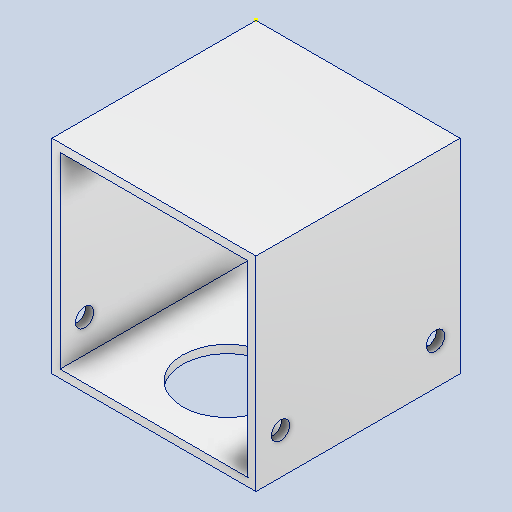
# Autodesk Inventor part: ankle
Saved by Autodesk Inventor 2022 (Build 260153000, 153)
## iProperties
Created: 2022-10-09
Part Number: ankle
Material: アルミニウム 6061
Document SubType Name: Modeling
Designer: haya
Density: 2.7 g/cm^3
Appearance: アルミニウム - フラット
Mass: 49.4438 g
Surface Area: 193.318 cm^2
Volume: 18.3125 cm^3
Author: haya
Autodesk Inventor part; units mm, degrees
ref_plane "YZ Plane" through (0, 0, 0) normal (1, 0, 0) x (0, 1, 0)
ref_plane "XZ Plane" through (0, 0, 0) normal (0, 1, 0) x (-1, 0, 0)
ref_plane "XY Plane" through (0, 0, 0) normal (0, 0, 1) x (1, 0, 0)
sketch "スケッチ1" plane through (0, 0, 0) normal (0, 0, 1) x (1, 0, 0)
  line L0 (0, 0) -> (50, 0)
  line L1 (50, 0) -> (50, 50)
  line L2 (50, 50) -> (0, 50)
  line L3 (0, 50) -> (0, 0)
  line L4 (2, 48) -> (48, 48)
  line L5 (48, 48) -> (48, 2)
  line L6 (48, 2) -> (2, 2)
  line L7 (2, 2) -> (2, 48)
  dimension "d0" = 50
  dimension "d1" = 2
  constraints: 16 end point, 4 parallel, 3 perpendicular, 1 horizontal, 3 other
  measures "d0" distance of L0.start L0.end
  measures "d1" distance between parallel lines of L4 L2
extrude "押し出し1" add sketch "スケッチ1" along normal blind 50
sketch "スケッチ2" plane through (0, 50, 0) normal (0, 1, 0) x (1, 0, 0)
  point P0 (0, 0)
sketch "スケッチ3" plane through (50, 0, 0) normal (1, 0, 0) x (0, 0, -1)
  line L0 (0, 0) -> (0, 50) projected
  line L1 (0, 50) -> (-50, 50) projected
  line L2 (-50, 0) -> (-50, 50) projected
  line L3 (0, 0) -> (-50, 0) projected
  line L4 (-50, 10) -> (0, 10) construction
  line L5 (-25, 50) -> (-25, 0) construction
  point P0 (-44, 10)
  point P1 (-6, 10)
  dimension "d5" = 6
  dimension "d21" = 10
  constraints: 4 end point, 3 point on line, 2 midpoint, 1 perpendicular, 1 symmetric about line
  measures "d5" distance from line of point (-44, 10) L2
  measures "d21" distance between parallel lines of L4 L3
hole "穴1" at (50, 10, 44) at (50, 10, 6) direction (-1, 0, 0) diameter 4.5 end through all
sketch "スケッチ4" plane through (0, 0, 0) normal (0, -1, 0) x (1, 0, 0)
  line L0 (0, 0) -> (50, 0) projected
  line L1 (50, 0) -> (50, 50) projected
  line L2 (0, 50) -> (50, 50) projected
  line L3 (0, 0) -> (0, 50) projected
  line L4 (25, 50) -> (25, 0) construction
  point P0 (25, 32)
  dimension "d20" = 18
  constraints: 2 end point, 2 midpoint, 1 point on line
  measures "d20" distance from line of point (25, 32) L2
hole "穴2" at (25, 0, 32) direction (0, 1, 0) diameter 22 depth 2
